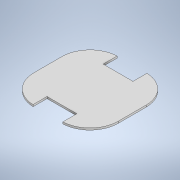
# Autodesk Inventor part: board_base
Saved by Autodesk Inventor 2020.3 (Build 243373000, 373)
## iProperties
Created: 2021-03-17
Part Number: board_base
Material: Ogólny
Document SubType Name: Modeling
Designer: patry
Density: 1 g/cm^3
Appearance: Domyślna
Author: patry
Autodesk Inventor part; units mm, degrees
ref_plane "YZ Plane" through (0, 0, 0) normal (1, 0, 0) x (0, 1, 0)
ref_plane "XZ Plane" through (0, 0, 0) normal (0, 1, 0) x (-1, 0, 0)
ref_plane "XY Plane" through (0, 0, 0) normal (0, 0, 1) x (1, 0, 0)
sketch "Szkic1" plane through (0, 0, 0) normal (0, 1, 0) x (-1, 0, 0)
  line L0 (15, 45) -> (-15, 45)
  line L1 (-45, 15) -> (-45, -15)
  line L2 (-15, -45) -> (15, -45)
  line L3 (45, -15) -> (45, 15)
  line L4 (45, 45) -> (-45, -45) construction
  line L5 (-45, 45) -> (45, -45) construction
  arc A0 (45, 43) -> (43, 45) centre (43, 43) ccw
  arc A1 (45, 15) -> (15, 45) centre (15, 15) ccw
  arc A2 (15, -45) -> (45, -15) centre (15, -15) ccw
  arc A3 (-45, -15) -> (-15, -45) centre (-15, -15) ccw
  arc A4 (-15, 45) -> (-45, 15) centre (-15, 15) ccw
  point P0 (0, 0)
  dimension "d0" = 90
  dimension "d1" = 90
  dimension "d3" = 30
  constraints: 12 end point, 10 point on circle, 10 point on line, 10 tangent, 5 centre point, 3 equal radius, 2 midpoint, 2 parallel, 1 horizontal, 1 perpendicular
  measures "d0" distance of L5.end L4.end
  measures "d1" distance of L4.end L5.start
  measures "d3" radius of A1
extrude "Wyciągnięcie proste1" add sketch "Szkic1" along normal blind 2
sketch "Szkic2" plane through (0, 2, 0) normal (0, 1, 0) x (1, 0, 0)
  line L0 (0, -49.4552) -> (0, 63.4462) construction
  line L1 (-44.5279, 0) -> (46.4745, 0) construction
  line L2 (16, 30) -> (-16, 30)
  line L3 (-16, 30) -> (-16, 45)
  line L4 (-16, 45) -> (16, 45)
  line L5 (16, 45) -> (16, 30)
  line L6 (16, 30) -> (-16, 45) construction
  line L7 (-16, 30) -> (16, 45) construction
  arc A0 (15, -45) -> (45, -15) centre (15, -15) ccw projected
  line L8 (45, -15) -> (45, 15) projected
  arc A1 (45, 15) -> (15, 45) centre (15, 15) ccw projected
  line L9 (15, 45) -> (-15, 45) projected
  arc A2 (-15, 45) -> (-45, 15) centre (-15, 15) ccw projected
  line L10 (-45, 15) -> (-45, -15) projected
  arc A3 (-45, -15) -> (-15, -45) centre (-15, -15) ccw projected
  line L11 (-15, -45) -> (15, -45) projected
  line L12 (15, 45) -> (-15, 45) projected
  line L13 (16, -45) -> (-16, -45)
  line L14 (-16, -45) -> (-16, -30)
  line L15 (-16, -30) -> (16, -30)
  line L16 (16, -30) -> (16, -45)
  line L17 (16, -45) -> (-16, -30) construction
  line L18 (-16, -45) -> (16, -30) construction
  line L19 (-15, -45) -> (15, -45) projected
  point P0 (0, 0)
  point P1 (0, 37.5)
  point P2 (0, -37.5)
  point P3 (0, -37.5)
  point P4 (0, 37.5)
  point P5 (-16, -40)
  point P6 (16, -40)
  dimension "d6" = 32
  dimension "d7" = 15
  dimension "d8" = 32
  dimension "d9" = 15
  constraints: 28 end point, 6 midpoint, 4 horizontal, 4 parallel, 2 collinear, 2 perpendicular, 2 vertical, 2 vertical alignment, 1 point on line
  measures "d6" distance of L3.end L4.end
  measures "d7" distance of L2.end L3.end
  measures "d8" distance of L15.start L15.end
  measures "d9" distance of L18.start L15.start
extrude "Wyciągnięcie proste2" cut sketch "Szkic2" against normal blind 10 contours L2 L3 A2 L4 A1 L5 | A1 L4 L5 | L3 L4 A2 | L16 L13 A0 | A0 L11 A3 L14 L15 L16 | A3 L13 L14
